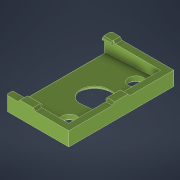
# Autodesk Inventor part: AdxlMount
Saved by Autodesk Inventor 2022.1 (Build 261234000, 234)
## iProperties
Created: 2021-08-06
Part Number: AdxlMount
Material: Generisch
Document SubType Name: Modeling
Designer: Rama
Density: 1 g/cm^3
Appearance: Olivgrün
Author: Rama
Autodesk Inventor part; units mm, degrees
ref_plane "YZ Plane" through (0, 0, 0) normal (1, 0, 0) x (0, 1, 0)
ref_plane "XZ Plane" through (0, 0, 0) normal (0, 1, 0) x (-1, 0, 0)
ref_plane "XY Plane" through (0, 0, 0) normal (0, 0, 1) x (1, 0, 0)
sketch "Skizze1" plane through (0, 0, 0) normal (0, 1, 0) x (-1, 0, 0)
  line L0 (8.15, 10.5) -> (-8.15, 10.5)
  line L1 (-8.15, 10.5) -> (-8.15, -10.5)
  line L2 (-8.15, -10.5) -> (8.15, -10.5)
  line L3 (8.15, -10.5) -> (8.15, 10.5)
  line L4 (8.15, 10.5) -> (-8.15, -10.5) construction
  line L5 (-8.15, 10.5) -> (8.15, -10.5) construction
  point P0 (0, 0)
  dimension "d0" = 16.3
  dimension "d1" = 21
  constraints: 12 end point, 2 midpoint, 2 parallel, 1 horizontal, 1 perpendicular
  measures "d0" distance of L2.end L1.end
  measures "d1" distance of L1.end L0.end
extrude "Extrusion1" add sketch "Skizze1" along normal blind 2
sketch "Skizze2" plane through (0, 2, 0) normal (0, 1, 0) x (1, 0, 0)
  line L0 (8.015, -10.27) -> (-8.015, -10.27)
  line L1 (-8.015, -10.27) -> (-8.015, 10.27)
  line L2 (-8.015, 10.27) -> (8.015, 10.27)
  line L3 (8.015, 10.27) -> (8.015, -10.27)
  line L4 (8.015, -10.27) -> (-8.015, 10.27) construction
  line L5 (-8.015, -10.27) -> (8.015, 10.27) construction
  line L6 (-8.015, 0) -> (5.335, 0)
  line L7 (5.335, 0) -> (5.335, -7.6)
  line L8 (5.335, 0) -> (12.935, 0) construction
  line L9 (5.335, -7.6) -> (5.335, 7.6)
  circle A0 centre (5.335, -7.6) radius 1.5
  circle A1 centre (5.335, 7.6) radius 1.5
  point P0 (0, 0)
  dimension "d4" = 16.03
  dimension "d5" = 20.54
  dimension "d6" = 13.35
  dimension "d7" = 7.6
  dimension "d8" = 90
  dimension "d9" = 15.2
  dimension "d10" = 3
  dimension "d11" = 3
  constraints: 20 end point, 3 horizontal, 3 midpoint, 2 centre point, 2 coincident, 2 parallel, 2 perpendicular, 1 point on line, 1 vertical
  measures "d4" distance of L1.end L2.end
  measures "d5" distance of L0.end L1.end
  measures "d6" distance of L6.start L6.end
  measures "d7" distance of L6.end L7.end
  measures "d8" angle of L7 L8
  measures "d9" distance of L7.end L9.end
  measures "d10" diameter of A0
  measures "d11" diameter of A1
extrude "Extrusion2" add sketch "Skizze2" along normal blind 2 contours A0 | A1
chamfer "Fase1" distance 0.5 angle 45 2 edges at (3.835, 4, -7.6) (3.835, 4, 7.6)
sketch "Skizze3" plane through (5.335, 4, -7.6) normal (0, 1, 0) x (1, 0, 0)
  line L0 (2.815, 2.9) -> (-13.485, 2.9) projected
  line L1 (2.815, -18.1) -> (-13.485, -18.1)
  line L2 (-13.485, -18.1) -> (-13.485, 2.9)
  line L3 (-13.485, 2.9) -> (2.815, 2.9)
  line L4 (2.815, 2.9) -> (2.815, -18.1)
  line L5 (2.815, -18.1) -> (-13.485, 2.9) construction
  line L6 (-13.485, -18.1) -> (2.815, 2.9) construction
  line L7 (4.315, -19.6) -> (-14.985, -19.6)
  line L8 (-14.985, -19.6) -> (-14.985, 4.4)
  line L9 (-14.985, 4.4) -> (4.315, 4.4)
  line L10 (4.315, 4.4) -> (4.315, -19.6)
  line L11 (4.315, -19.6) -> (-14.985, 4.4) construction
  line L12 (-14.985, -19.6) -> (4.315, 4.4) construction
  point P0 (-5.335, -7.6)
  dimension "d17" = 19.3
  dimension "d18" = 24
  constraints: 24 end point, 4 midpoint, 4 parallel, 2 horizontal, 2 perpendicular
  measures "d17" distance of L8.end L9.end
  measures "d18" distance of L7.end L8.end
extrude "Extrusion3" add sketch "Skizze3" against normal up to surface (4 mm away)
sketch "Skizze4" plane through (0, 0, 0) normal (0, -1, 0) x (1, 0, 0)
  line L0 (-9.65, 12) -> (-9.65, -12) projected
  line L1 (-9.65, -12) -> (9.65, -12) projected
  line L2 (9.65, -12) -> (9.65, 12) projected
  line L3 (9.65, 12) -> (-9.65, 12) projected
  point P0 (0, 0)
extrude "Extrusion4" cut sketch "Skizze4" against normal blind 1
sketch "Skizze5" plane through (0, 2, 0) normal (0, 1, 0) x (1, 0, 0)
  line L0 (-8.15, -10.5) -> (8.15, -10.5) projected
  line L1 (-8.15, 10.5) -> (-4.65, 10.5)
  line L2 (-4.65, 10.5) -> (-4.65, -10.5)
  line L3 (-4.65, -10.5) -> (-8.15, -10.5)
  line L4 (-8.15, -10.5) -> (-8.15, 10.5)
  point P0 (0, 0)
  dimension "d23" = 3.5
  constraints: 8 end point, 2 parallel, 1 horizontal, 1 perpendicular, 1 point on line
  measures "d23" distance of L2.end L3.end
extrude "Extrusion5" cut sketch "Skizze5" against normal through all
sketch "Skizze6" plane through (8.15, 4, 10.5) normal (0, 0, -1) x (-1, 0, 0)
  line L0 (0, 0) -> (16.3, 0) projected
  line L1 (8.15, 0) -> (8.15, -0.3)
  line L2 (8.15, 0) -> (8.45, 0) construction
  line L3 (8.15, -0.3) -> (8.15, 0.5)
  line L4 (6.65, -0.3) -> (9.65, -0.3)
  line L5 (9.65, -0.3) -> (9.65, 0.5)
  line L6 (9.65, 0.5) -> (6.65, 0.5)
  line L7 (6.65, 0.5) -> (6.65, -0.3)
  line L8 (6.65, -0.3) -> (9.65, 0.5) construction
  line L9 (9.65, -0.3) -> (6.65, 0.5) construction
  point P0 (8.15, -4)
  point P1 (8.15, 0.1)
  dimension "d26" = 0.3
  dimension "d27" = 90
  dimension "d28" = 0.8
  dimension "d29" = 3
  dimension "d30" = 0.8
  constraints: 18 end point, 4 midpoint, 2 horizontal, 2 parallel, 2 perpendicular, 1 point on line, 1 vertical
  measures "d26" distance of L1.start L1.end
  measures "d27" angle of L1 L2
  measures "d28" distance of L1.end L3.end
  measures "d29" distance of L6.end L5.end
  measures "d30" distance of L5.end L4.end
extrude "Extrusion6" add sketch "Skizze6" along normal blind 0.8
sketch "Skizze7" plane through (8.15, 4, 10.5) normal (0, 0, 1) x (1, 0, 0)
  line L0 (-6.65, 0) -> (-9.65, 0) projected
  line L1 (-6.65, 0.5) -> (-6.65, 0) projected
  line L2 (-9.65, 0.5) -> (-6.65, 0.5) projected
  line L3 (-9.65, 0) -> (-9.65, 0.5) projected
  point P0 (-8.15, -4)
extrude "Extrusion7" add sketch "Skizze7" along normal up to surface (1.5 mm away)
chamfer "Fase2" distance 0.5 angle 45 2 edges at (1.5, 4, 11.25) (-1.5, 4, 11.25)
chamfer "Fase4" distance 0.6 angle 45 1 edges at (0, 4.5, 9.7)
fillet "Rundung3" radius 0.3 2 edges at (0, 3.7, 9.7) (0, 3.9, 9.7)
sketch "Skizze8" plane through (8.15, 4, -10.5) normal (-1, 0, 0) x (0, 0, 1)
  line L0 (0, 0) -> (21, 0) projected
  line L1 (10.5, 0) -> (10.5, -0.3)
  line L2 (10.5, -0.3) -> (12, -0.3)
  line L3 (12, -0.3) -> (12, 0.5)
  line L4 (12, 0.5) -> (10.5, 0.5)
  line L5 (10.5, 0.5) -> (10.5, -0.3)
  line L6 (10.5, -0.3) -> (9, -0.3)
  line L7 (9, -0.3) -> (9, 0.5)
  line L8 (9, 0.5) -> (10.5, 0.5)
  line L9 (10.5, 0.5) -> (10.5, -0.3)
  point P0 (10.5, -4)
  point P1 (10.5, 0.5)
  dimension "d47" = 0.3
  dimension "d48" = 1.5
  dimension "d49" = 0.8
  dimension "d50" = 1.5
  constraints: 18 end point, 4 parallel, 2 horizontal, 2 perpendicular, 1 midpoint, 1 point on line, 1 vertical
  measures "d47" distance of L1.start L1.end
  measures "d48" distance of L4.end L3.end
  measures "d49" distance of L3.end L2.end
  measures "d50" distance of L7.end L8.end
extrude "Extrusion8" add sketch "Skizze8" along normal blind 0.8
chamfer "Fase5" distance 0.6 angle 45 1 edges at (7.35, 4.5, 0)
fillet "Rundung4" radius 0.3 2 edges at (7.35, 3.7, 0) (7.35, 3.9, 0)
sketch "Skizze9" plane through (8.15, 4, -10.5) normal (1, 0, 0) x (0, 0, -1)
  line L0 (-9, 0) -> (-12, 0) projected
  line L1 (-9, 0.5) -> (-9, 0) projected
  line L2 (-12, 0.5) -> (-9, 0.5) projected
  line L3 (-12, 0) -> (-12, 0.5) projected
  point P0 (-10.5, -4)
extrude "Extrusion9" add sketch "Skizze9" along normal up to surface (1.5 mm away)
chamfer "Fase6" distance 0.5 angle 45 2 edges at (8.9, 4, 1.5) (8.9, 4, -1.5)
sketch "Skizze10" plane through (-8.15, 4, -10.5) normal (0, 0, 1) x (1, 0, 0)
  line L0 (0, 0) -> (16.3, 0) projected
  line L1 (3.5, 0) -> (5.5, 0)
  line L2 (5.5, 0) -> (5.5, -0.3)
  line L3 (5.5, -0.3) -> (3.5, -0.3)
  line L4 (3.5, -0.3) -> (3.5, 0)
  line L5 (3.5, 0) -> (5.5, 0)
  line L6 (5.5, 0) -> (5.5, 0.5)
  line L7 (5.5, 0.5) -> (3.5, 0.5)
  line L8 (3.5, 0.5) -> (3.5, 0)
  point P0 (8.15, -4)
  dimension "d62" = 2
  dimension "d63" = 0.3
  dimension "d64" = 2
  dimension "d65" = 0.5
  constraints: 16 end point, 4 parallel, 2 horizontal, 2 perpendicular, 1 point on line
  measures "d62" distance of L2.end L3.end
  measures "d63" distance of L1.end L2.end
  measures "d64" distance of L7.end L6.end
  measures "d65" distance of L6.end L5.end
extrude "Extrusion10" add sketch "Skizze10" along normal blind 0.8
sketch "Skizze11" plane through (-8.15, 4, -10.5) normal (0, 0, -1) x (-1, 0, 0)
  line L0 (-3.5, 0) -> (-5.5, 0) projected
  line L1 (-3.5, 0.5) -> (-3.5, 0) projected
  line L2 (-5.5, 0.5) -> (-3.5, 0.5) projected
  line L3 (-5.5, 0) -> (-5.5, 0.5) projected
  point P0 (-8.15, -4)
extrude "Extrusion11" add sketch "Skizze11" along normal up to surface (1.5 mm away)
chamfer "Fase7" distance 0.5 angle 45 2 edges at (-2.65, 4, -11.25) (-4.65, 4, -11.25)
chamfer "Fase8" distance 0.6 angle 45 1 edges at (-3.65, 4.5, -9.7)
fillet "Rundung6" radius 0.3 2 edges at (-3.65, 3.9, -9.7) (-3.65, 3.7, -9.7)
chamfer "Fase9" distance 0.2 angle 45 3 edges at (-3.65, 3.7, -10.5) (8.15, 3.7, 0) (0, 3.7, 10.5)
fillet "Rundung7" radius 1 3 edges at (0, 3.7, 10.3) (7.95, 3.7, 0) (-3.65, 3.7, -10.3)
ref_plane "Arbeitsebene1" through (0, -0.5, 0) normal (0, -1, 0) x (1, 0, 0)
sketch "Skizze14" plane through (0, -0.5, 0) normal (0, -1, 0) x (1, 0, 0)
  circle A0 centre (3.55, 0) radius 4
  point P0 (0, 0)
  constraints: 1 centre point
extrude "Extrusion14" cut sketch "Skizze14" against normal through all
sketch "Skizze15" plane through (5.335, 4, 7.6) normal (0, 1, 0) x (1, 0, 0)
  line L0 (-9.985, 18.1) -> (-9.985, -2.9)
  line L1 (-9.985, -2.9) -> (2.815, -2.9)
  line L2 (2.815, -2.9) -> (2.815, 18.1)
  line L3 (2.815, 18.1) -> (-9.985, 18.1)
  circle A0 centre (0, 15.2) radius 1.5
  circle A1 centre (0, 0) radius 1.5
  point P0 (-5.335, 7.6)
  constraints: 8 end point, 4 centre point
extrude "Extrusion15" cut sketch "Skizze15" against normal up to surface (2 mm away) contours A0 | A1
hole "Bohrung2" at (5.335, 4, 7.6) at (5.335, 4, -7.6) direction (0, -1, 0) diameter 3.3 end through all clearance for "Innensechskantkopfschraube" size "M3" standard "ANSI Metrisches M Profil"
sketch "Skizze17" plane through (5.335, 4, -7.6) normal (0, 1, 0) x (1, 0, 0)
  line L0 (-13.485, 2.9) -> (-13.485, -18.1) projected
  line L1 (-13.485, -18.1) -> (-15, -18.1)
  line L2 (-15, -18.1) -> (-15, 2.9)
  line L3 (-15, 2.9) -> (-13.485, 2.9)
  line L4 (-13.485, 2.9) -> (-13.485, -18.1)
  point P0 (-5.335, -7.6)
  constraints: 8 end point, 2 parallel, 1 horizontal, 1 perpendicular
extrude "Extrusion16" cut sketch "Skizze17" against normal up to surface (2 mm away)
sketch "Skizze18" plane through (0, 2, 0) normal (0, 1, 0) x (1, 0, 0)
  circle A0 centre (5.335, 7.6) radius 1.2295 projected
  circle A1 centre (5.335, -7.6) radius 1.2295 projected
  line L0 (-13.05, -9.55) -> (13.05, -9.55) projected
  line L1 (13.05, -9.55) -> (13.05, 9.55) projected
  line L2 (13.05, 9.55) -> (-13.05, 9.55) projected
  line L3 (-13.05, 9.55) -> (-13.05, -9.55) projected
  circle A2 centre (3.55, 0) radius 4 projected
  line L4 (-9.65, -10.5) -> (-9.65, 10.5) projected
  line L5 (-8.15, -10.5) -> (-9.65, -10.5) projected
  line L6 (-8.15, 10.5) -> (-8.15, -10.5) projected
  line L7 (-9.65, 10.5) -> (-8.15, 10.5) projected
  line L8 (-8.15, 10.5) -> (-8.15, -10.5) projected
  line L9 (-8.15, 0) -> (-10.85, 0)
  line L10 (-8.15, 0) -> (-5.45, 0) construction
  circle A3 centre (-10.85, 0) radius 2.7
  line L11 (-9.65, -10.5) -> (-9.65, 10.5) projected
  line L12 (-9.65, -9.55) -> (-13.05, -1.5652)
  line L13 (-9.65, 9.55) -> (-13.05, 1.5652)
  point P0 (0, 0)
  dimension "d111" = 2.7
  dimension "d112" = 180
  dimension "d113" = 5.4
  constraints: 8 end point, 6 point on line, 2 point on circle, 1 centre point, 1 coincident, 1 collinear, 1 horizontal, 1 midpoint, 1 perpendicular
  measures "d111" distance of L9.start L9.end
  measures "d112" angle of L9 L10
  measures "d113" diameter of A3
sketch "Skizze19" plane through (5.335, 4, -7.6) normal (0, 1, 0) x (1, 0, 0)
  line L0 (4.315, 4.4) -> (-14.985, 4.4) projected
  line L1 (-14.985, -19.6) -> (-9.985, -19.6)
  line L2 (-9.985, -19.6) -> (-9.985, 4.4)
  line L3 (-9.985, 4.4) -> (-14.985, 4.4)
  line L4 (-14.985, 4.4) -> (-14.985, -19.6)
  point P0 (-5.335, -7.6)
  dimension "d123" = 5
  constraints: 8 end point, 2 parallel, 1 horizontal, 1 perpendicular, 1 point on line
  measures "d123" distance of L3.end L2.end
extrude "Extrusion18" cut sketch "Skizze19" against normal through all both and the other way through all
sketch "Skizze20" plane through (0, 1, 0) normal (0, -1, 0) x (1, 0, 0)
  line L0 (-4.65, 12) -> (-4.65, -12) projected
  line L1 (9.65, -12) -> (-4.65, -12) projected
  line L2 (9.65, 12) -> (9.65, -12) projected
  line L3 (-4.65, 12) -> (9.65, 12) projected
  circle A0 centre (5.335, 7.6) radius 1.65 projected
  circle A1 centre (5.335, -7.6) radius 1.65 projected
  circle A2 centre (3.55, 0) radius 4 projected
  point P0 (0, 0)
extrude "Extrusion19" add sketch "Skizze20" along normal blind 0.5
sketch "Skizze21" plane through (0, 2, 0) normal (0, 1, 0) x (1, 0, 0)
  circle A0 centre (5.335, -7.6) radius 1.65 projected
  circle A1 centre (5.335, 7.6) radius 1.65 projected
  circle A2 centre (3.55, 0) radius 4 projected
  line L0 (-4.65, 10.5) -> (-4.65, -10.5) projected
  line L1 (-4.65, -10.5) -> (8.15, -10.5) projected
  line L2 (8.15, -10.5) -> (8.15, 10.5) projected
  line L3 (8.15, 10.5) -> (-4.65, 10.5) projected
  circle A3 centre (3.55, 0) radius 1.8
  point P0 (0, 0)
  dimension "d128" = 3.6
  constraints: 1 centre point, 1 coincident
  measures "d128" diameter of A3
extrude "Extrusion20" add sketch "Skizze21" against normal blind 0.5 contours A2
sketch "Skizze22" plane through (0, 0.5, 0) normal (0, -1, 0) x (1, 0, 0)
  circle A0 centre (3.55, 0) radius 4 projected
  circle A1 centre (3.55, 0) radius 1.8 projected
  circle A2 centre (3.55, 0) radius 4 projected
  line L0 (3.55, -4) -> (9.65, -4)
  line L1 (9.65, -12) -> (9.65, 12) projected
  line L2 (3.55, 4) -> (9.65, 4)
  line L3 (9.65, 12) -> (9.65, 2) projected
  line L4 (9.65, 4) -> (9.65, -4)
  point P0 (0, 0)
  constraints: 6 end point, 2 point on line, 1 horizontal, 1 parallel, 1 perpendicular, 1 vertical alignment, 3 other
extrude "Extrusion21" cut sketch "Skizze22" against normal up to surface (1 mm away) contours A0 L2 L1 L0
sketch "Skizze23" plane through (0, 1.5, 0) normal (0, -1, 0) x (1, 0, 0)
  arc A0 (3.55, 4) -> (3.55, -4) centre (3.55, 0) ccw projected
  line L0 (3.55, -4) -> (9.65, -4) projected
  line L1 (9.65, 4) -> (9.65, -4) projected
  line L2 (9.65, 4) -> (3.55, 4) projected
  circle A1 centre (3.55, 0) radius 1.8 projected
  point P0 (0, 0)
extrude "Extrusion22" add sketch "Skizze23" against normal blind 1
sketch "Skizze24" plane through (0, 1.5, 0) normal (0, -1, 0) x (1, 0, 0)
  arc A0 (3.55, 4) -> (3.55, -4) centre (3.55, 0) ccw projected
  line L0 (3.55, -4) -> (9.65, -4) projected
  line L1 (9.65, 4) -> (9.65, -4) projected
  line L2 (9.65, 4) -> (3.55, 4) projected
  circle A1 centre (3.55, 0) radius 1.8 projected
  point P0 (0, 0)
extrude "Extrusion23" cut sketch "Skizze24" against normal blind 0.5
sketch "Skizze25" plane through (0, 2.5, 0) normal (0, 1, 0) x (1, 0, 0)
  line L0 (8.15, 4) -> (8.15, -4) projected
  line L1 (8.15, 4) -> (3.55, 4) projected
  arc A0 (3.55, 4) -> (3.55, -4) centre (3.55, 0) ccw projected
  line L2 (3.55, -4) -> (8.15, -4) projected
  circle A1 centre (3.55, 0) radius 1.8 projected
  circle A2 centre (3.55, 0) radius 4.5
  line L3 (8.15, 10.5) -> (8.15, 2) projected
  line L4 (3.55, -4.5) -> (8.15, -4.5)
  line L5 (8.15, -4.5) -> (8.15, 4.5)
  line L6 (8.15, 4.5) -> (3.55, 4.5)
  line L7 (3.55, 4.5) -> (3.55, -4.5)
  point P0 (0, 0)
  dimension "d137" = 9
  constraints: 8 end point, 2 parallel, 1 coincident, 1 horizontal, 1 perpendicular, 1 point on line, 3 other
extrude "Extrusion24" add sketch "Skizze25" against normal blind 0.5 contours L1 A2 L6 L3 | L1 L7 A2 | L5 L4 A2 L2 | A0 L7 A2 | A2 L7 L2
chamfer "Fase11" distance 1.5 angle 45 3 edges at (6.6, 2, -4) (-0.45, 2, 0) (6.6, 2, 4)
sketch "Skizze26" plane through (0, 2.5, 0) normal (0, 1, 0) x (1, 0, 0)
  line L0 (8.15, 4.5) -> (8.15, -4.5) projected
  line L1 (8.15, 4.5) -> (3.55, 4.5) projected
  arc A0 (3.55, 4.5) -> (3.55, -4.5) centre (3.55, 0) ccw projected
  line L2 (3.55, -4.5) -> (8.15, -4.5) projected
  circle A1 centre (3.55, 0) radius 1.8 projected
  point P0 (0, 0)
extrude "Extrusion25" cut sketch "Skizze26" against normal blind 0.5
sketch "Skizze27" plane through (9.65, 4, -2) normal (1, 0, 0) x (0, 0, -1)
  line L0 (-4.5, -2) -> (-6, -3.5) projected
  line L1 (-4.5, -2) -> (0.5, -2) projected
  line L2 (2, -3.5) -> (0.5, -2) projected
  line L3 (10, -3.5) -> (2, -3.5) projected
  line L4 (10, 0) -> (10, -3.5) projected
  line L5 (0, 0) -> (10, 0) projected
  line L6 (-0.5, 0.5) -> (0, 0) projected
  line L7 (-3.5, 0.5) -> (-0.5, 0.5) projected
  line L8 (-4, 0) -> (-3.5, 0.5) projected
  line L9 (-14, 0) -> (-4, 0) projected
  line L10 (-14, 0) -> (-14, -3.5) projected
  line L11 (-6, -3.5) -> (-14, -3.5) projected
  line L12 (-14, -3.5) -> (10, -3.5) projected
  line L13 (-14, 0) -> (-4, 0) projected
  line L14 (10, -3.5) -> (-14, -3.5)
  line L15 (-14, -3.5) -> (-14, 0)
  line L16 (-14, 0) -> (10, 0)
  line L17 (10, 0) -> (10, -3.5)
  point P0 (-2, -4)
  constraints: 8 end point, 2 parallel, 1 horizontal, 1 perpendicular
extrude "Extrusion26" add sketch "Skizze27" against normal up to surface (1.5 mm away) contours L1 L2 L12 L0
fillet "Rundung10" radius 2 2 edges at (8.15, 1.25, 3.25) (8.15, 1.25, -3.25)
sketch "Skizze28" plane through (8.15, 2, -10.5) normal (0, 0, 1) x (1, 0, 0)
  line L0 (0, 0) -> (-12.8, 0) projected
  line L1 (0, 2) -> (0, 0) projected
  line L2 (0, 0) -> (-12.8, -0.7829)
  line L3 (-12.8, 2.5) -> (-12.8, -1.5) projected
  line L4 (0, 0) -> (12.8239, 0) construction
  point P0 (-8.15, -2)
  dimension "d150" = 176.5
  constraints: 4 end point, 1 equal length, 1 horizontal, 1 point on line
  measures "d150" angle of L2 L4
extrude "Extrusion27" cut sketch "Skizze28" along normal up to surface (21 mm away)
fillet "Rundung12" radius 0.1 5 edges at (4.85, 1.7982, 2.7019) (7.4798, 1.959, 1.8253) (4.85, 1.7982, -2.7019) (7.4798, 1.959, -1.8253) (0.5873, 1.5374, 0)
fillet "Rundung13" radius 0.3 2 edges at (-4.65, 1.2171, 0) (-4.65, 0.5, 0)
chamfer "Fase12" distance 0.3 angle 45 7 edges at (2.65, 0.5, -12) (-4.5621, 0.5879, -12) (-4.65, 2.65, -12) (9.65, 0.5, 0) (2.65, 0.5, 12) (-4.5621, 0.5879, 12) (-4.65, 2.4, 12)
chamfer "Fase13" distance 0.2 angle 45 2 edges at (3.685, 0.5, 7.6) (3.685, 0.5, -7.6)
